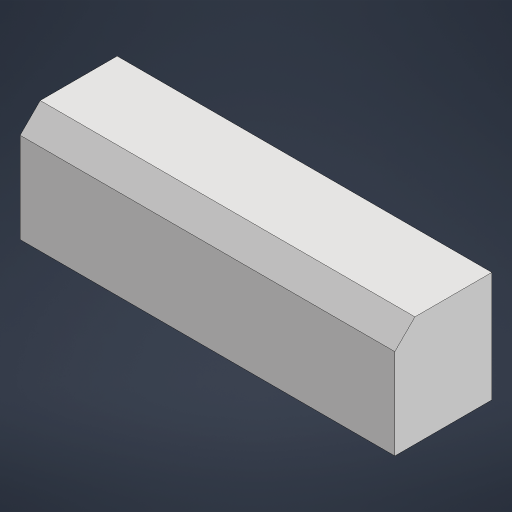
# Autodesk Inventor part: Wall_cap
Saved by Autodesk Inventor 2023.1 (Build 271208000, 208)
## iProperties
Created: 2022-11-19
Part Number: Wall_cap
Material: Generic
Document SubType Name: Modeling
Designer: awelt
Mass: 3366.01 g
Surface Area: 1549.63 cm^2
Volume: 3366.01 cm^3
Density: 1 g/cm^3
Appearance: Default
RuleStatus: InUse
BeforeDocSave0: file://C:\Users\awelt\Documents\Inventor\iLogic_Rules\BoundingStore
DocClose0: file://C:\Users\awelt\Documents\Inventor\iLogic_Rules\BoundingStore
Author: awelt
BoundingBL1: 3 5/8
BoundingBL2: 4 1/8
BoundingBL3: 14
BoundingCF: 0.121
Autodesk Inventor part; units mm, degrees
ref_plane "YZ Plane" through (0, 0, 0) normal (1, 0, 0) x (0, 1, 0)
ref_plane "XZ Plane" through (0, 0, 0) normal (0, 1, 0) x (-1, 0, 0)
ref_plane "XY Plane" through (0, 0, 0) normal (0, 0, 1) x (1, 0, 0)
sketch "Sketch2" plane through (0, 0, 0) normal (1, 0, 0) x (0, 1, 0)
  line L0 (0, 0) -> (0, 92.075)
  line L1 (0, 0) -> (104.775, 0)
  line L2 (104.775, 0) -> (104.775, 73.025)
  line L3 (0, 92.075) -> (85.725, 92.075)
  line L4 (104.775, 73.025) -> (85.725, 92.075)
  dimension "d3" = 92.075
  dimension "d4" = 104.775
  dimension "d5" = 73.025
  dimension "d6" = 85.725
  constraints: 10 end point, 2 horizontal, 1 perpendicular, 1 vertical
  measures "d3" distance of L0.start L0.end
  measures "d4" distance of L0.start L1.end
  measures "d5" distance of L1.end L2.end
  measures "d6" distance of L0.end L3.end
extrude "Extrusion1" add sketch "Sketch2" along normal blind 355.6
body "Solid1"
